Autodesk Inventor part; units mm, degrees
(part 2 of 2)
sketch "Sketch12" plane through (0, 0, 2.55) normal (0, 0, 1) x (1, 0, 0)
  line L0 (1.7095, -0.3755) -> (1.8711, -0.3755)
  line L1 (1.7095, -0.8624) -> (1.7095, -0.3755)
  line L2 (1.7111, -0.0516) -> (1.7111, -0.2119)
  line L3 (1.5448, -0.0527) -> (1.7096, -0.0527)
  line L4 (1.5467, -0.0514) -> (1.5467, -0.2124)
  line L5 (1.5462, -0.2119) -> (1.5462, -0.3755)
  line L6 (1.3838, -0.0514) -> (1.5467, -0.0514)
  line L7 (1.3838, -0.2124) -> (1.3838, -0.0514)
  line L8 (0.8919, -0.3755) -> (0.8919, -0.2124)
  line L9 (1.221, -0.0527) -> (1.0581, -0.0527)
  line L10 (1.056, -0.3755) -> (0.8919, -0.3755)
  line L11 (1.056, -0.2124) -> (1.056, -0.3755)
  line L12 (0.8919, -0.2124) -> (1.056, -0.2124)
  line L13 (1.8711, -0.3755) -> (1.8711, -0.0516)
  line L14 (1.8711, -0.5378) -> (1.8711, -0.3755)
  line L15 (2.0309, -0.5378) -> (1.8711, -0.5378)
  line L16 (1.8711, -0.3755) -> (2.1907, -0.3755)
  line L17 (2.1907, -0.3755) -> (2.1907, -0.5378)
  line L18 (2.1907, -0.3755) -> (2.1907, -0.0491)
  line L19 (2.1907, -0.0491) -> (2.3485, -0.0491)
  line L20 (2.3485, -0.0491) -> (2.3485, -0.3755)
  line L21 (2.3485, -0.3755) -> (2.1907, -0.3755)
  line L22 (1.5467, -0.2124) -> (1.3838, -0.2124)
  line L23 (1.2209, -0.3755) -> (1.057, -0.3755)
  line L24 (1.2209, -0.5378) -> (1.2209, -0.3755)
  line L25 (1.057, -0.7023) -> (0.8965, -0.7023)
  line L26 (1.057, -0.3755) -> (1.057, -0.7023)
  line L27 (1.384, -0.3755) -> (1.384, -0.5378)
  line L28 (1.5462, -0.3755) -> (1.384, -0.3755)
  line L29 (1.7111, -0.2119) -> (1.5462, -0.2119)
  line L30 (1.384, -0.5378) -> (1.2209, -0.5378)
  line L31 (0.8965, -0.7023) -> (0.8965, -1.024)
  line L32 (1.384, -0.7023) -> (1.384, -0.5378)
  line L33 (1.384, -0.5378) -> (1.5462, -0.5378)
  line L34 (1.0586, -1.024) -> (1.0586, -0.8624)
  line L35 (1.5462, -0.5378) -> (1.5462, -0.7023)
  line L36 (1.5462, -0.7023) -> (1.384, -0.7023)
  line L37 (1.0586, -0.8624) -> (1.7095, -0.8624)
  line L38 (0.4096, -0.2124) -> (0.5728, -0.2124)
  line L39 (0.5728, -0.2124) -> (0.5728, -0.3755)
  line L40 (0.5728, -0.0514) -> (0.7344, -0.0514)
  line L41 (0.4096, -0.3755) -> (0.4096, -0.2124)
  line L42 (0.5728, -0.3755) -> (0.4096, -0.3755)
  line L43 (0.4096, -1.0246) -> (0.4096, -0.8624)
  line L44 (0.4096, -0.8624) -> (0.5728, -0.8624)
  line L45 (0.5728, -0.8624) -> (0.5728, -0.7031)
  line L46 (0.5728, -0.7031) -> (0.8961, -0.7031)
  line L47 (0.8961, -0.7031) -> (0.8961, -0.5378)
  line L48 (0.8961, -0.5378) -> (0.4096, -0.5378)
  line L49 (2.1907, -0.5378) -> (2.3485, -0.5378)
  line L50 (2.0309, -0.7023) -> (2.0309, -0.5378)
  line L51 (2.1907, -0.7023) -> (2.0309, -0.7023)
  line L52 (2.3485, -0.5378) -> (2.3485, -1.0249)
  line L53 (2.1907, -1.0249) -> (2.1907, -0.7023)
  line L54 (2.3485, -1.0249) -> (2.1907, -1.0249)
  line L55 (2.0328, -0.8624) -> (2.0328, -1.024)
  line L56 (2.1907, -1.024) -> (2.0328, -1.024)
  line L57 (0.8919, -1.6707) -> (1.056, -1.6707)
  line L58 (1.2181, -1.6707) -> (1.2181, -1.5065)
  line L59 (1.3818, -1.6707) -> (1.2181, -1.6707)
  line L60 (1.2181, -1.5065) -> (1.3818, -1.5065)
  line L61 (1.3818, -1.5065) -> (1.3818, -1.6707)
  line L62 (0.8961, -1.1813) -> (1.2209, -1.1813)
  line L63 (0.8965, -1.024) -> (1.0586, -1.024)
  line L64 (1.2209, -1.1813) -> (1.2209, -1.024)
  line L65 (1.2209, -1.024) -> (1.5448, -1.024)
  line L66 (1.5448, -1.024) -> (1.5448, -1.1813)
  line L67 (1.7075, -1.5065) -> (1.7075, -1.6707)
  line L68 (1.5448, -1.1813) -> (1.7095, -1.1813)
  line L69 (1.7075, -1.6707) -> (1.8711, -1.6707)
  line L70 (1.8711, -1.6707) -> (1.8711, -1.5065)
  line L71 (1.8711, -1.5065) -> (1.7075, -1.5065)
  line L72 (0.8961, -1.3385) -> (1.8711, -1.3385)
  line L73 (1.8711, -1.5065) -> (2.0329, -1.5065)
  line L74 (2.1907, -1.5065) -> (2.0329, -1.5065)
  line L75 (2.3485, -1.6707) -> (2.3485, -1.345)
  line L76 (2.3485, -1.345) -> (2.1907, -1.345)
  line L77 (2.1907, -1.345) -> (2.1907, -1.5065)
  line L78 (1.8711, -1.3385) -> (1.8711, -1.5065)
  line L79 (2.0329, -1.5065) -> (2.0329, -1.3385)
  line L80 (2.0329, -1.3385) -> (1.8711, -1.3385)
  line L81 (1.8711, -1.1813) -> (1.8711, -1.3385)
  line L82 (1.8711, -1.1813) -> (2.1907, -1.1813)
  line L83 (1.7095, -1.1813) -> (1.7095, -0.8624)
  line L84 (1.7095, -0.8624) -> (2.0328, -0.8624)
  line L85 (2.1907, -1.024) -> (2.1907, -1.1813)
  line L86 (0.7344, -1.8284) -> (0.7344, -1.994)
  line L87 (0.7344, -1.994) -> (0.5728, -1.994)
  line L88 (0.5728, -1.8284) -> (0.7344, -1.8284)
  line L89 (0.5728, -1.8284) -> (0.5728, -1.6643)
  line L90 (0.2544, -2.154) -> (0.4096, -2.154)
  line L91 (1.056, -2.1533) -> (0.8919, -2.1533)
  line L92 (0.4096, -2.154) -> (0.4096, -1.8284)
  line L93 (0.5728, -1.994) -> (0.5728, -1.8284)
  line L94 (0.8919, -2.1533) -> (0.8919, -1.6707)
  line L95 (1.056, -1.6707) -> (1.056, -2.1533)
  line L96 (0.4096, -1.8284) -> (0.5728, -1.8284)
  line L97 (1.5448, -2.642) -> (1.5448, -2.1533)
  line L98 (2.0329, -1.5065) -> (2.0329, -1.6707)
  line L99 (1.5448, -2.1533) -> (2.035, -2.1533)
  line L100 (1.3838, -2.8055) -> (1.3838, -1.9925)
  line L101 (1.3838, -1.9925) -> (2.1893, -1.9925)
  line L102 (2.0329, -1.6707) -> (2.3485, -1.6707)
  line L103 (2.035, -2.1533) -> (2.035, -2.642)
  line L104 (2.035, -2.642) -> (1.5448, -2.642)
  line L105 (1.2202, -1.8269) -> (2.3506, -1.8269)
  line L106 (2.1893, -1.9925) -> (2.1893, -2.8055)
  line L107 (2.1893, -2.8055) -> (1.3838, -2.8055)
  line L108 (2.3506, -1.8269) -> (2.3506, -2.9562)
  line L109 (2.3506, -2.9562) -> (1.2202, -2.9562)
  line L110 (1.2202, -2.9562) -> (1.2202, -1.8269)
  line L111 (0.4102, -2.3154) -> (0.5779, -2.3154)
  line L112 (0.7355, -2.3134) -> (1.0581, -2.3134)
  line L113 (1.0581, -2.4698) -> (0.8968, -2.4698)
  line L114 (1.0581, -2.3134) -> (1.0581, -2.4698)
  line L115 (0.5779, -2.4774) -> (0.4102, -2.4774)
  line L116 (0.5779, -2.3154) -> (0.5779, -2.4774)
  line L117 (0.8968, -2.4698) -> (0.8968, -2.6397)
  line L118 (0.8968, -2.6397) -> (0.7355, -2.6397)
  line L119 (0.7355, -2.6397) -> (0.7355, -2.3134)
  line L120 (0.4102, -2.4774) -> (0.4102, -2.3154)
  line L121 (0.4102, -2.6397) -> (0.7355, -2.6397)
  line L122 (0.4102, -2.8009) -> (0.4102, -2.6397)
  line L123 (0.5728, -2.8009) -> (0.4102, -2.8009)
  line L124 (0.7355, -2.9621) -> (0.7355, -2.6397)
  line L125 (0.7355, -2.9621) -> (0.5728, -2.9621)
  line L126 (0.4102, -2.8009) -> (0.255, -2.8009)
  line L127 (0.4102, -2.8009) -> (0.4102, -2.9622)
  line L128 (0.4102, -2.9622) -> (0.0925, -2.9622)
  line L129 (0.5728, -2.9621) -> (0.5728, -2.8009)
  line L130 (0.5728, -1.5065) -> (0.4096, -1.5065)
  line L131 (0.7355, -1.0246) -> (0.4096, -1.0246)
  line L132 (0.4096, -1.1892) -> (0.5728, -1.1892)
  line L133 (0.7355, -1.3385) -> (0.7355, -1.0246)
  line L134 (0.8961, -1.3385) -> (0.8961, -1.1813)
  line L135 (0.8961, -1.3385) -> (0.7355, -1.3385)
  line L136 (0.4096, -1.5065) -> (0.4096, -1.1892)
  line L137 (0.5728, -1.1892) -> (0.5728, -1.5065)
  line L138 (0.7355, -1.5014) -> (0.8961, -1.5014)
  line L139 (0.5728, -1.6643) -> (0.7355, -1.6643)
  line L140 (0.7355, -1.6643) -> (0.7355, -1.5014)
  line L141 (0.8961, -1.5014) -> (0.8961, -1.3385)
  line L142 (-0.0746, -0.8624) -> (-0.2282, -0.8624)
  line L143 (-0.2342, -0.7031) -> (-0.0746, -0.7031)
  line L144 (-0.0746, -0.7031) -> (-0.0746, -0.5378)
  line L145 (-0.2342, -0.5378) -> (-0.2342, -0.7031)
  line L146 (-0.0746, -0.5378) -> (-0.2342, -0.5378)
  line L147 (-0.0746, -0.3755) -> (-0.0746, -0.5378)
  line L148 (-0.5577, -0.7031) -> (-0.3973, -0.7031)
  line L149 (-0.3973, -0.3755) -> (-0.3973, -0.5378)
  line L150 (-0.5577, -0.5378) -> (-0.5577, -0.7031)
  line L151 (-0.3973, -0.5378) -> (-0.5577, -0.5378)
  line L152 (-0.0746, -0.7031) -> (-0.0746, -0.8624)
  line L153 (-0.2282, 0.2745) -> (-0.2282, -0.0491)
  line L154 (-0.2282, -0.0491) -> (-0.0746, -0.0491)
  line L155 (-0.0746, -0.0491) -> (-0.0746, -0.2124)
  line L156 (-0.0746, -0.2124) -> (-0.2282, -0.2124)
  line L157 (-0.2282, -0.2124) -> (-0.2282, -0.0491)
  line L158 (-0.2282, -0.0491) -> (-0.3967, -0.0491)
  line L159 (-0.0746, -0.3755) -> (-0.2357, -0.3755)
  line L160 (-0.5566, 0.1109) -> (-0.3967, 0.1109)
  line L161 (-0.2357, -0.3755) -> (-0.2357, -0.2124)
  line L162 (-0.5566, 0.1109) -> (-0.5566, -0.0491)
  line L163 (-0.2357, -0.2124) -> (-0.5577, -0.2124)
  line L164 (-0.3973, -0.3755) -> (-0.5577, -0.3755)
  line L165 (-0.3967, -0.0491) -> (-0.3967, 0.1109)
  line L166 (0.2535, -1.6707) -> (0.0919, -1.6707)
  line L167 (0.0919, -1.8284) -> (0.2544, -1.8284)
  line L168 (0.2535, -1.5065) -> (0.2535, -1.6707)
  line L169 (0.0919, -1.5065) -> (0.2535, -1.5065)
  line L170 (0.0919, -1.6707) -> (0.0919, -1.5065)
  line L171 (0.0919, -1.1813) -> (0.2507, -1.1813)
  line L172 (-0.2357, -1.8284) -> (-0.0711, -1.8284)
  line L173 (-0.2357, -1.6643) -> (-0.2357, -1.8284)
  line L174 (-0.3973, -1.8284) -> (-0.2342, -1.8284)
  line L175 (-0.3973, -1.8284) -> (-0.3973, -1.6643)
  line L176 (0.0919, -1.3385) -> (0.0919, -1.5064)
  line L177 (0.0919, -1.5064) -> (-0.2342, -1.5064)
  line L178 (-0.0711, -1.3385) -> (0.0919, -1.3385)
  line L179 (-0.3973, -1.6643) -> (-0.2357, -1.6643)
  line L180 (-0.2342, -1.5064) -> (-0.2342, -1.3385)
  line L181 (-0.0711, -1.1813) -> (-0.0711, -1.3385)
  line L182 (-0.3973, -1.1813) -> (-0.0711, -1.1813)
  line L183 (-0.2342, -1.3385) -> (-0.3973, -1.3385)
  line L184 (-0.3973, -1.3385) -> (-0.3973, -1.5014)
  line L185 (-0.7175, -0.3755) -> (-0.7175, -0.7001)
  line L186 (-0.5577, -0.2124) -> (-0.5577, -0.3755)
  line L187 (-0.8836, -0.7001) -> (-0.8836, -0.5378)
  line L188 (-0.8836, -0.3755) -> (-0.7175, -0.3755)
  line L189 (-0.5566, -0.0491) -> (-1.0463, -0.0491)
  line L190 (-0.8836, -0.2124) -> (-0.8836, -0.3755)
  line L191 (-0.8836, -0.5378) -> (-1.0463, -0.5378)
  line L192 (-1.0463, -0.5378) -> (-1.0463, -0.3755)
  line L193 (-1.2063, -0.537) -> (-1.2063, -0.7001)
  line L194 (-1.2063, -0.7001) -> (-1.3676, -0.7001)
  line L195 (-1.3676, -0.537) -> (-1.2063, -0.537)
  line L196 (-1.3676, -0.7001) -> (-1.3676, -0.537)
  line L197 (-1.3676, -0.3755) -> (-1.0463, -0.3755)
  line L198 (-1.3676, -0.3755) -> (-1.3676, -0.2124)
  line L199 (-0.7175, -0.7001) -> (-0.8836, -0.7001)
  line L200 (-0.5566, 0.1109) -> (-0.7175, 0.1109)
  line L201 (-0.5566, 0.2726) -> (-0.5566, 0.1109)
  line L202 (-0.7175, 0.2726) -> (-0.5566, 0.2726)
  line L203 (-0.7175, 0.1109) -> (-0.7175, 0.2726)
  line L204 (-1.0463, -0.0491) -> (-1.0463, -0.2124)
  line L205 (-1.0463, -0.2124) -> (-0.8836, -0.2124)
  line L206 (-1.0463, 0.1109) -> (-0.8836, 0.1109)
  line L207 (-0.8836, 0.1109) -> (-0.8836, 0.4344)
  line L208 (-1.0463, 0.2726) -> (-1.0463, 0.1109)
  line L209 (-1.2069, 0.2726) -> (-1.0463, 0.2726)
  line L210 (-1.2069, 0.1115) -> (-1.2069, 0.2726)
  line L211 (-1.2069, -0.2124) -> (-1.2069, -0.0491)
  line L212 (-1.3676, -0.2124) -> (-1.2069, -0.2124)
  line L213 (-1.3676, -0.0491) -> (-1.3676, 0.1115)
  line L214 (-1.2069, -0.0491) -> (-1.3676, -0.0491)
  line L215 (-1.208, 0.4384) -> (-1.208, 0.2726)
  line L216 (-1.3676, 0.1115) -> (-1.2069, 0.1115)
  line L217 (-1.208, 0.2726) -> (-1.6886, 0.2726)
  line L218 (-1.208, 0.4384) -> (-1.8491, 0.4384)
  line L219 (-1.528, -0.2124) -> (-1.528, -0.0491)
  line L220 (-1.528, -0.0491) -> (-1.6886, -0.0491)
  line L221 (-1.8491, -0.2124) -> (-1.528, -0.2124)
  line L222 (-1.2069, -1.3385) -> (-1.2069, -1.5014)
  line L223 (-1.2069, -1.5014) -> (-1.528, -1.5014)
  line L224 (-1.0463, -1.5014) -> (-1.0463, -1.6643)
  line L225 (-1.528, -1.6643) -> (-1.0463, -1.6643)
  line L226 (-1.528, -1.5014) -> (-1.528, -1.6643)
  line L227 (-1.3682, -1.3385) -> (-1.2069, -1.3385)
  line L228 (-1.0463, -1.3385) -> (-1.0463, -1.1856)
  line L229 (-1.0463, -1.1856) -> (-1.3682, -1.1856)
  line L230 (-1.3682, -1.1856) -> (-1.3682, -1.3385)
  line L231 (-1.528, -1.1856) -> (-1.3682, -1.1856)
  line L232 (-1.3682, -1.1856) -> (-1.3682, -1.024)
  line L233 (-1.3682, -1.024) -> (-1.0463, -1.024)
  line L234 (-1.6826, -0.8624) -> (-1.6826, -1.3385)
  line L235 (-1.528, -0.8624) -> (-1.528, -1.1856)
  line L236 (-1.0463, -0.8624) -> (-1.528, -0.8624)
  line L237 (-1.0463, -1.024) -> (-1.0463, -0.8624)
  line L238 (-0.3973, -0.7031) -> (-0.3973, -1.1813)
  line L239 (-0.7181, -0.8624) -> (-0.8825, -0.8624)
  line L240 (-0.8825, -0.8624) -> (-0.8825, -1.024)
  line L241 (-0.8825, -1.024) -> (-1.0463, -1.024)
  line L242 (-1.0463, -1.1856) -> (-0.7181, -1.1856)
  line L243 (-0.7181, -1.1856) -> (-0.7181, -0.8624)
  line L244 (-1.0463, -1.024) -> (-1.0463, -1.1856)
  line L245 (-2.1731, -0.0514) -> (-2.3367, -0.0514)
  line L246 (-2.3367, -0.0514) -> (-2.3367, 0.1105)
  line L247 (-2.3367, 0.1105) -> (-2.1731, 0.1105)
  line L248 (-2.0121, -0.0491) -> (-1.8491, -0.0491)
  line L249 (-2.1731, 0.1105) -> (-2.1731, -0.0514)
  line L250 (-2.0121, 0.1109) -> (-2.0121, -0.0491)
  line L251 (-1.6886, -0.0491) -> (-1.6886, 0.2726)
  line L252 (-2.0121, 0.2745) -> (-2.174, 0.2745)
  line L253 (-2.174, 0.2745) -> (-2.174, 0.4344)
  line L254 (-2.174, 0.4344) -> (-2.0121, 0.4344)
  line L255 (-2.0121, 0.4344) -> (-2.0121, 0.2745)
  line L256 (-1.8491, 0.4384) -> (-1.8491, 0.1109)
  line L257 (-1.8491, 0.1109) -> (-2.0121, 0.1109)
  line L258 (0.4096, 0.1105) -> (0.4096, 0.2745)
  line L259 (-0.0705, 0.4344) -> (-0.0705, 0.2745)
  line L260 (-0.0705, 0.2745) -> (-0.2282, 0.2745)
  line L261 (-0.0705, 0.4344) -> (0.2555, 0.4344)
  line L262 (0.2555, 0.2745) -> (0.2555, 0.4344)
  line L263 (0.4096, 0.2745) -> (0.2555, 0.2745)
  line L264 (0.4096, 0.4344) -> (0.4096, 0.2745)
  line L265 (-1.8491, -0.0491) -> (-1.8491, -0.2124)
  line L266 (-2.1731, -0.2124) -> (-2.0121, -0.2124)
  line L267 (-2.0121, -0.2124) -> (-2.0121, -0.3755)
  line L268 (-2.1731, -0.3755) -> (-2.1731, -0.2124)
  line L269 (-2.0121, -0.3755) -> (-2.1731, -0.3755)
  line L270 (-2.0099, -0.5378) -> (-2.0099, -0.3755)
  line L271 (-2.0099, -0.3755) -> (-1.6886, -0.3755)
  line L272 (-1.6886, -0.3755) -> (-1.6886, -0.5378)
  line L273 (-2.3339, -0.7001) -> (-2.3339, -0.5378)
  line L274 (-2.0069, -0.7001) -> (-2.3339, -0.7001)
  line L275 (-1.6886, -0.5378) -> (-1.8481, -0.5378)
  line L276 (-2.1731, -0.8624) -> (-2.0069, -0.8624)
  line L277 (-2.0069, -0.8624) -> (-2.0069, -0.7001)
  line L278 (-1.8481, -0.5378) -> (-1.8481, -0.8624)
  line L279 (-1.8481, -0.8624) -> (-1.6826, -0.8624)
  line L280 (-2.1731, -1.1856) -> (-2.1731, -0.8624)
  line L281 (-2.3339, -0.5378) -> (-2.0099, -0.5378)
  line L282 (-0.0746, -0.5378) -> (0.0919, -0.5378)
  line L283 (0.0919, -0.3755) -> (0.0919, -0.5378)
  line L284 (0.4096, -0.5378) -> (0.4096, -0.3755)
  line L285 (0.4096, -0.3755) -> (0.0919, -0.3755)
  line L286 (0.0919, -0.7031) -> (-0.0746, -0.7031)
  line L287 (0.0919, -0.7031) -> (0.0919, -0.8624)
  line L288 (-0.2282, -0.8624) -> (-0.2282, -1.0246)
  line L289 (-0.2282, -1.0246) -> (0.0919, -1.0246)
  line L290 (0.2507, -0.8624) -> (0.0919, -0.8624)
  line L291 (0.0919, -1.0246) -> (0.0919, -1.1813)
  line L292 (0.2507, -1.1813) -> (0.2507, -0.8624)
  line L293 (-1.8457, -1.3385) -> (-1.8457, -1.1856)
  line L294 (-1.6826, -1.3385) -> (-1.8457, -1.3385)
  line L295 (-1.6886, -1.5065) -> (-1.6886, -1.6707)
  line L296 (-2.0121, -1.5065) -> (-1.6886, -1.5065)
  line L297 (-1.6886, -1.6707) -> (-2.0121, -1.6707)
  line L298 (-1.8457, -1.1856) -> (-2.0121, -1.1856)
  line L299 (-2.0121, -1.6707) -> (-2.0121, -1.5065)
  line L300 (-2.0121, -1.1856) -> (-2.0121, -1.3385)
  line L301 (-2.0121, -1.3385) -> (-2.1731, -1.3385)
  line L302 (-2.1731, -1.3385) -> (-2.1731, -1.6643)
  line L303 (-2.3367, -1.1856) -> (-2.1731, -1.1856)
  line L304 (-2.3367, -1.6643) -> (-2.3367, -1.1856)
  line L305 (-2.1731, -1.6643) -> (-2.3367, -1.6643)
  line L306 (-0.7181, -1.3385) -> (-0.7181, -1.1856)
  line L307 (-0.7181, -1.1856) -> (-0.3973, -1.1856)
  line L308 (-0.3973, -1.1856) -> (-0.3973, -1.3385)
  line L309 (-0.7181, -1.5014) -> (-0.7181, -1.3385)
  line L310 (-0.3973, -1.3385) -> (-0.7181, -1.3385)
  line L311 (-0.7175, -1.8284) -> (-0.7175, -1.9925)
  line L312 (-0.7175, -1.9925) -> (-0.5577, -1.9925)
  line L313 (-0.5577, -1.9925) -> (-0.5577, -1.8284)
  line L314 (-0.5577, -1.8284) -> (-0.7175, -1.8284)
  line L315 (-0.3973, -1.9925) -> (-0.3973, -1.8284)
  line L316 (-0.5577, -1.6643) -> (-0.7181, -1.6643)
  line L317 (-0.5577, -1.6643) -> (-0.5577, -1.8284)
  line L318 (-0.5577, -1.8284) -> (-0.3973, -1.8284)
  line L319 (-0.7181, -1.5014) -> (-0.7181, -1.6643)
  line L320 (-0.3973, -1.5014) -> (-0.7181, -1.5014)
  line L321 (-0.7181, -1.8284) -> (-0.7181, -1.6643)
  line L322 (-1.0463, -1.3385) -> (-0.7181, -1.3385)
  line L323 (-1.0463, -1.5014) -> (-0.7181, -1.5014)
  line L324 (-0.7181, -1.6643) -> (-1.0463, -1.6643)
  line L325 (-0.8827, -1.9925) -> (-0.8827, -1.8284)
  line L326 (-0.8827, -1.8284) -> (-0.7181, -1.8284)
  line L327 (-1.0463, -1.6643) -> (-1.0463, -1.9925)
  line L328 (-0.8827, -1.9925) -> (-0.7175, -1.9925)
  line L329 (-0.7175, -1.9925) -> (-0.7175, -2.1533)
  line L330 (-0.7175, -2.1533) -> (-0.8827, -2.1533)
  line L331 (-0.8827, -2.1533) -> (-0.8827, -1.9925)
  line L332 (-1.0463, -1.9925) -> (-0.8827, -1.9925)
  line L333 (-0.3967, -2.1533) -> (-0.3967, -2.3123)
  line L334 (-0.7175, -2.1533) -> (-0.3967, -2.1533)
  line L335 (-0.7175, -2.1533) -> (-0.7175, -2.4774)
  line L336 (-1.0463, -2.3154) -> (-0.8827, -2.3154)
  line L337 (-0.7175, -2.4774) -> (-0.8827, -2.4774)
  line L338 (-0.8827, -2.3154) -> (-0.8827, -2.4774)
  line L339 (-1.0463, -2.4774) -> (-1.0463, -2.3154)
  line L340 (-0.8827, -2.4774) -> (-1.0463, -2.4774)
  line L341 (-0.8827, -2.4774) -> (-0.8827, -2.642)
  line L342 (-2.174, -1.9925) -> (-1.3685, -1.9925)
  line L343 (-2.3376, -1.8269) -> (-1.2073, -1.8269)
  line L344 (-2.013, -2.642) -> (-2.013, -2.1533)
  line L345 (-2.174, -2.8055) -> (-2.174, -1.9925)
  line L346 (-1.5228, -2.1533) -> (-1.5228, -2.642)
  line L347 (-1.5228, -2.642) -> (-2.013, -2.642)
  line L348 (-2.3376, -2.9562) -> (-2.3376, -1.8269)
  line L349 (-1.3685, -1.9925) -> (-1.3685, -2.8055)
  line L350 (-1.3685, -2.8055) -> (-2.174, -2.8055)
  line L351 (-1.2073, -1.8269) -> (-1.2073, -2.9562)
  line L352 (-1.2073, -2.9562) -> (-2.3376, -2.9562)
  line L353 (-2.013, -2.1533) -> (-1.5228, -2.1533)
  line L354 (-1.0463, -2.642) -> (-0.8827, -2.642)
  line L355 (-0.3967, -2.642) -> (-0.3967, -2.8009)
  line L356 (-0.3967, -2.8009) -> (-0.5571, -2.8009)
  line L357 (-0.5571, -2.642) -> (-0.3967, -2.642)
  line L358 (-0.5571, -2.8009) -> (-0.5571, -2.642)
  line L359 (-0.3967, -2.8009) -> (-0.3967, -2.9644)
  line L360 (-0.7175, -2.642) -> (-0.7175, -2.8009)
  line L361 (-0.7175, -2.8009) -> (-0.8827, -2.8009)
  line L362 (-0.8827, -2.642) -> (-0.7175, -2.642)
  line L363 (-0.8827, -2.8009) -> (-0.8827, -2.642)
  line L364 (-0.3967, -2.9644) -> (-1.0463, -2.9644)
  line L365 (-1.0463, -2.9644) -> (-1.0463, -2.642)
  line L366 (-0.0682, -2.3123) -> (-0.0682, -2.154)
  line L367 (-0.0711, -2.154) -> (0.0919, -2.154)
  line L368 (0.255, -2.8009) -> (0.255, -2.4774)
  line L369 (0.0925, -2.9622) -> (0.0925, -2.8009)
  line L370 (-0.3967, -2.3123) -> (-0.2351, -2.3123)
  line L371 (-0.2351, -2.154) -> (-0.2351, -2.3123)
  line L372 (-0.2351, -2.8009) -> (-0.3967, -2.8009)
  line L373 (-0.2351, -2.642) -> (-0.2351, -2.8009)
  line L374 (-0.0705, -2.642) -> (-0.2351, -2.642)
  line L375 (-0.2351, -2.3123) -> (-0.2351, -2.4774)
  line L376 (-0.2351, -2.3123) -> (-0.0682, -2.3123)
  line L377 (-0.0682, -2.154) -> (-0.2351, -2.154)
  line L378 (0.0925, -2.8009) -> (-0.0705, -2.8009)
  line L379 (-0.2351, -2.4774) -> (0.255, -2.4774)
  line L380 (-0.0705, -2.8009) -> (-0.0705, -2.642)
  line L381 (0.2544, -1.8284) -> (0.2544, -2.154)
  line L382 (0.0919, -2.154) -> (0.0919, -1.8284)
  line L383 (-0.0711, -1.8284) -> (-0.0711, -2.154)
  line L384 (-0.2342, -1.8284) -> (-0.2342, -1.9925)
  line L385 (-0.2342, -1.9925) -> (-0.3973, -1.9925)
  line L386 (0.5728, 0.1105) -> (0.4096, 0.1105)
  line L387 (0.4096, 0.2745) -> (0.5728, 0.2745)
  line L388 (0.894, 0.4344) -> (0.5779, 0.4344)
  line L389 (0.735, 0.6007) -> (0.4102, 0.6007)
  line L390 (0.735, 0.6007) -> (0.735, 0.7514)
  line L391 (0.735, 0.7514) -> (0.894, 0.7514)
  line L392 (0.4102, 0.9146) -> (0.894, 0.9146)
  line L393 (0.894, 0.7514) -> (0.894, 0.4344)
  line L394 (1.0581, 0.4344) -> (1.0581, 0.9141)
  line L395 (1.0581, 0.4344) -> (1.5448, 0.4344)
  line L396 (1.2202, 0.6007) -> (1.2202, 0.7514)
  line L397 (1.3818, 0.6007) -> (1.2202, 0.6007)
  line L398 (1.2202, 0.7514) -> (1.3818, 0.7514)
  line L399 (1.3818, 0.7514) -> (1.3818, 0.6007)
  line L400 (0.5728, 1.239) -> (0.5728, 1.0768)
  line L401 (0.894, 1.0768) -> (1.3838, 1.0768)
  line L402 (0.894, 0.9146) -> (0.894, 1.0768)
  line L403 (0.7345, 1.0768) -> (0.7345, 1.239)
  line L404 (0.7345, 1.239) -> (1.2209, 1.239)
  line L405 (0.7345, 1.4023) -> (0.7345, 1.239)
  line L406 (0.5728, 1.0768) -> (0.7345, 1.0768)
  line L407 (0.7345, 1.239) -> (0.5728, 1.239)
  line L408 (0.5728, 1.4023) -> (0.7345, 1.4023)
  line L409 (0.5728, 1.5644) -> (0.5728, 1.4023)
  line L410 (1.2209, 1.5644) -> (0.5728, 1.5644)
  line L411 (1.2209, 1.239) -> (1.2209, 1.5644)
  line L412 (0.0919, 1.5644) -> (0.2507, 1.5644)
  line L413 (0.0919, 1.4017) -> (0.0919, 1.5644)
  line L414 (0.2507, 1.239) -> (0.2507, 1.5644)
  line L415 (-0.0733, 1.5644) -> (-0.0733, 1.4017)
  line L416 (0.2507, 1.0768) -> (0.2507, 1.239)
  line L417 (-0.2353, 1.5644) -> (-0.0733, 1.5644)
  line L418 (0.2507, 1.239) -> (-0.2353, 1.239)
  line L419 (-0.2353, 1.239) -> (-0.2353, 1.5644)
  line L420 (0.2507, 1.73) -> (-0.3973, 1.73)
  line L421 (-0.3973, 1.73) -> (-0.3973, 1.0768)
  line L422 (-0.0733, 1.4017) -> (0.0919, 1.4017)
  line L423 (0.7344, 0.1105) -> (0.5728, 0.1105)
  line L424 (0.5728, 0.2745) -> (0.5728, 0.1105)
  line L425 (0.894, 0.2745) -> (0.894, 0.1115)
  line L426 (0.5779, 0.2745) -> (0.894, 0.2745)
  line L427 (0.5779, 0.4344) -> (0.5779, 0.2745)
  line L428 (1.0581, 0.2745) -> (1.3838, 0.2745)
  line L429 (1.3838, 0.2745) -> (1.3838, 0.1115)
  line L430 (1.3838, 0.1115) -> (1.5448, 0.1115)
  line L431 (1.5448, 0.1115) -> (1.5448, -0.0527)
  line L432 (1.0581, 0.1115) -> (1.0581, 0.2745)
  line L433 (1.0581, 0.1115) -> (1.221, 0.1115)
  line L434 (1.221, 0.1115) -> (1.221, -0.0527)
  line L435 (1.0581, -0.0527) -> (1.0581, 0.1115)
  line L436 (0.7344, -0.0514) -> (0.7344, 0.1105)
  line L437 (0.5728, 0.1105) -> (0.5728, -0.0514)
  line L438 (0.894, 0.1115) -> (1.0581, 0.1115)
  line L439 (1.3838, 1.0768) -> (1.3838, 1.2402)
  line L440 (1.5462, 1.4023) -> (1.5462, 1.5644)
  line L441 (1.5448, 0.9141) -> (1.0581, 0.9141)
  line L442 (1.5467, 1.2402) -> (1.5467, 1.0768)
  line L443 (1.5462, 1.4023) -> (1.7111, 1.4023)
  line L444 (1.7096, 1.0768) -> (1.7096, 0.9141)
  line L445 (1.3838, 1.2402) -> (1.5467, 1.2402)
  line L446 (1.7096, 0.2745) -> (1.7096, -0.0527)
  line L447 (1.8711, -0.0516) -> (1.7111, -0.0516)
  line L448 (1.8711, 0.2745) -> (1.8711, 0.1117)
  line L449 (2.0328, 0.1117) -> (2.0328, -0.0491)
  line L450 (2.0328, -0.0491) -> (2.1907, -0.0491)
  line L451 (2.1907, -0.0491) -> (2.1907, 0.2745)
  line L452 (2.1907, 0.2745) -> (1.8711, 0.2745)
  line L453 (1.8711, 0.1117) -> (2.0328, 0.1117)
  line L454 (1.5467, 1.0768) -> (1.7096, 1.0768)
  line L455 (2.0302, 0.4343) -> (2.1838, 0.4343)
  line L456 (1.8711, 0.2745) -> (1.7096, 0.2745)
  line L457 (1.8711, 0.6015) -> (1.8711, 0.2745)
  line L458 (2.1838, 0.4343) -> (2.1838, 0.5928)
  line L459 (2.0302, 0.6015) -> (2.0302, 0.4343)
  line L460 (2.0302, 0.6015) -> (1.8711, 0.6015)
  line L461 (2.1838, 0.7546) -> (2.1838, 0.5928)
  line L462 (1.7096, 0.7514) -> (1.8711, 0.7514)
  line L463 (1.5448, 0.9141) -> (1.5448, 0.4344)
  line L464 (1.8711, 0.9141) -> (2.0302, 0.9141)
  line L465 (1.8711, 0.7514) -> (1.8711, 0.9141)
  line L466 (1.7096, 0.7514) -> (1.7096, 0.9141)
  line L467 (2.0302, 0.9141) -> (2.0302, 0.7546)
  line L468 (2.0302, 0.7546) -> (2.1838, 0.7546)
  line L469 (0.4102, 0.9141) -> (0.4102, 1.0768)
  line L470 (0.4102, 1.0768) -> (0.2507, 1.0768)
  line L471 (0.2555, 0.4344) -> (0.4096, 0.4344)
  line L472 (0.2555, 0.4344) -> (0.2555, 0.6023)
  line L473 (0.4102, 0.6007) -> (0.4102, 0.9146)
  line L474 (-0.0702, 0.6023) -> (0.2555, 0.6023)
  line L475 (-0.0702, 0.7535) -> (-0.0702, 0.6023)
  line L476 (-0.0733, 0.9141) -> (0.4102, 0.9141)
  line L477 (-0.2351, 0.7535) -> (-0.0702, 0.7535)
  line L478 (-0.2351, 0.6023) -> (-0.2351, 0.7535)
  line L479 (-0.3946, 0.6023) -> (-0.2351, 0.6023)
  line L480 (-0.0733, 1.0768) -> (-0.0733, 0.9141)
  line L481 (-0.3973, 1.0768) -> (-0.0733, 1.0768)
  line L482 (1.7111, 1.0832) -> (1.7111, 1.4023)
  line L483 (2.0309, 1.2402) -> (2.0309, 1.0832)
  line L484 (2.0309, 1.0832) -> (1.7111, 1.0832)
  line L485 (1.8711, 1.4023) -> (1.8711, 1.2402)
  line L486 (1.7111, 1.73) -> (1.7111, 1.5644)
  line L487 (1.8711, 1.2402) -> (2.0309, 1.2402)
  line L488 (2.1907, 1.4023) -> (1.8711, 1.4023)
  line L489 (1.7111, 1.5644) -> (2.3485, 1.5644)
  line L490 (2.3485, 1.2402) -> (2.1907, 1.2402)
  line L491 (2.3485, 1.5644) -> (2.3485, 1.2402)
  line L492 (2.1907, 1.2402) -> (2.1907, 1.4023)
  line L493 (0.2507, 1.5644) -> (0.2507, 1.73)
  line L494 (0.4102, 1.239) -> (0.2507, 1.239)
  line L495 (0.4102, 1.5644) -> (0.4102, 1.239)
  line L496 (0.2507, 1.5644) -> (0.4102, 1.5644)
  line L497 (0.4102, 1.73) -> (0.4102, 1.5644)
  line L498 (0.5728, 1.5644) -> (0.5728, 1.73)
  line L499 (0.5728, 1.73) -> (0.4102, 1.73)
  line L500 (0.4102, 1.5644) -> (0.5728, 1.5644)
  line L501 (-0.8836, 0.4344) -> (-1.0463, 0.4344)
  line L502 (-1.0463, 0.4344) -> (-1.0463, 0.9141)
  line L503 (-0.8827, 0.6023) -> (-0.7175, 0.6023)
  line L504 (-0.7175, 0.6023) -> (-0.7175, 0.7514)
  line L505 (-0.7175, 0.7514) -> (-0.8827, 0.7514)
  line L506 (-0.5544, 0.7514) -> (-0.7175, 0.7514)
  line L507 (-0.5544, 0.7514) -> (-0.5544, 0.9141)
  line L508 (-0.7175, 0.7514) -> (-0.7175, 1.0768)
  line L509 (-0.3946, 0.9141) -> (-0.3946, 0.6023)
  line L510 (-0.5544, 0.9141) -> (-0.3946, 0.9141)
  line L511 (-1.0463, 1.0768) -> (-1.0463, 1.2402)
  line L512 (-1.0463, 1.4036) -> (-1.0463, 1.2402)
  line L513 (-0.8827, 0.7514) -> (-0.8827, 0.6023)
  line L514 (-0.7175, 1.0768) -> (-0.5566, 1.0768)
  line L515 (-0.8836, 0.9141) -> (-0.8836, 1.0768)
  line L516 (-1.0463, 0.9141) -> (-0.8836, 0.9141)
  line L517 (-0.5566, 1.0768) -> (-0.5566, 1.4036)
  line L518 (-0.7175, 1.2402) -> (-0.8827, 1.2402)
  line L519 (-0.7175, 1.4036) -> (-0.7175, 1.2402)
  line L520 (-0.8836, 1.0768) -> (-1.0463, 1.0768)
  line L521 (-0.5566, 1.4036) -> (-0.5566, 1.5644)
  line L522 (-0.8827, 1.4036) -> (-0.7175, 1.4036)
  line L523 (-0.8827, 1.5644) -> (-0.5566, 1.5644)
  line L524 (-0.8827, 1.4036) -> (-0.8827, 1.5644)
  line L525 (-1.0463, 1.4036) -> (-0.8827, 1.4036)
  line L526 (-0.8827, 1.2402) -> (-0.8827, 1.4036)
  line L527 (-0.8836, 1.5644) -> (-1.0463, 1.5644)
  line L528 (-0.8836, 1.73) -> (-0.8836, 1.5644)
  line L529 (-1.0463, 1.73) -> (-0.8836, 1.73)
  line L530 (-1.0463, 1.5644) -> (-1.0463, 1.73)
  line L531 (1.2209, 1.5644) -> (1.2209, 1.73)
  line L532 (1.5462, 1.5644) -> (1.2209, 1.5644)
  line L533 (1.2209, 1.73) -> (1.7111, 1.73)
  line L534 (1.2374, 2.5034) -> (1.3667, 2.5034)
  line L535 (1.3667, 2.5034) -> (1.3667, 2.2334)
  line L536 (1.3667, 2.2334) -> (1.2374, 2.2334)
  line L537 (1.2374, 2.6356) -> (1.2374, 2.5034)
  line L538 (0.8281, 2.6356) -> (1.2374, 2.6356)
  line L539 (1.2374, 2.5034) -> (0.8281, 2.5034)
  line L540 (1.2374, 2.2334) -> (1.2374, 2.5034)
  line L541 (1.2374, 2.2334) -> (0.8281, 2.2334)
  line L542 (1.2374, 2.109) -> (1.2374, 2.2334)
  line L543 (0.8281, 2.109) -> (1.2374, 2.109)
  line L544 (0.8281, 2.6356) -> (0.6989, 2.6356)
  line L545 (0.8281, 2.5034) -> (0.8281, 2.6356)
  line L546 (0.8281, 2.2334) -> (0.8281, 2.109)
  line L547 (0.8281, 2.5034) -> (0.8281, 2.2334)
  line L548 (0.6989, 2.2334) -> (0.6989, 2.5034)
  line L549 (0.6989, 2.5034) -> (0.8281, 2.5034)
  line L550 (0.5437, 2.2334) -> (0.5437, 2.109)
  line L551 (0.8281, 2.2334) -> (0.6989, 2.2334)
  line L552 (-1.5219, 1.4036) -> (-1.5219, 0.9149)
  line L553 (-1.3676, 1.5644) -> (-1.3676, 0.7514)
  line L554 (-1.5219, 0.9149) -> (-2.0121, 0.9149)
  line L555 (-2.0121, 1.4036) -> (-1.5219, 1.4036)
  line L556 (-2.0121, 0.9149) -> (-2.0121, 1.4036)
  line L557 (-1.2063, 1.73) -> (-1.2063, 0.6007)
  line L558 (-1.3676, 0.7514) -> (-2.1731, 0.7514)
  line L559 (-2.1731, 1.5644) -> (-1.3676, 1.5644)
  line L560 (-1.2063, 0.6007) -> (-2.3367, 0.6007)
  line L561 (-2.3367, 0.6007) -> (-2.1731, 0.6007)
  line L562 (-2.1731, 0.7514) -> (-2.1731, 1.5644)
  line L563 (-2.3367, 0.6007) -> (-2.3367, 1.73)
  line L564 (-2.3367, 1.73) -> (-1.2063, 1.73)
  line L565 (-1.3676, 2.2334) -> (-1.5014, 2.2334)
  line L566 (-1.5014, 2.2334) -> (-1.5014, 2.109)
  line L567 (-1.0999, 2.2334) -> (-1.2274, 2.2334)
  line L568 (-1.0999, 2.109) -> (-1.0999, 2.2334)
  line L569 (-1.5014, 2.109) -> (-1.0999, 2.109)
  line L570 (-0.1284, 2.7689) -> (-0.1284, 2.9022)
  line L571 (0.0138, 2.7689) -> (-0.1284, 2.7689)
  line L572 (-0.1284, 2.9022) -> (0.0138, 2.9022)
  line L573 (0.0138, 2.9022) -> (0.0138, 2.7689)
  line L574 (0.0138, 3.0367) -> (0.0138, 2.9022)
  line L575 (0.2766, 2.5034) -> (0.143, 2.5034)
  line L576 (0.2766, 2.6356) -> (0.2766, 2.5034)
  line L577 (0.4102, 2.6356) -> (0.4102, 2.9022)
  line L578 (0.4102, 2.6356) -> (0.2766, 2.6356)
  line L579 (0.2766, 2.5034) -> (0.4102, 2.5034)
  line L580 (0.4102, 2.5034) -> (0.4102, 2.6356)
  line L581 (0.0138, 2.9022) -> (0.4102, 2.9022)
  line L582 (0.4102, 2.9022) -> (0.4102, 3.0367)
  line L583 (0.4102, 3.0367) -> (0.0138, 3.0367)
  line L584 (0.8281, 2.9022) -> (0.8281, 2.6356)
  line L585 (0.6989, 2.9022) -> (0.8281, 2.9022)
  line L586 (0.6989, 2.6356) -> (0.6989, 2.9022)
  line L587 (0.5437, 2.9022) -> (0.5437, 2.6356)
  line L588 (0.4102, 2.9022) -> (0.5437, 2.9022)
  line L589 (0.5437, 2.6356) -> (0.4102, 2.6356)
  line L590 (-0.2763, 3.0367) -> (-0.2763, 2.109)
  line L591 (0.2766, 2.3684) -> (0.2766, 2.5034)
  line L592 (0.143, 2.3684) -> (0.2766, 2.3684)
  line L593 (0.5437, 2.109) -> (-0.1284, 2.109)
  line L594 (-0.1284, 2.2334) -> (0.5437, 2.2334)
  line L595 (0.143, 2.2334) -> (0.143, 2.3684)
  line L596 (0.143, 2.5034) -> (0.143, 2.3684)
  line L597 (0.0138, 2.2334) -> (0.143, 2.2334)
  line L598 (0.143, 2.3684) -> (0.0138, 2.3684)
  line L599 (0.0138, 2.3684) -> (0.0138, 2.2334)
  line L600 (-0.1284, 2.109) -> (-0.1284, 2.2334)
  line L601 (-0.4137, 2.109) -> (-0.4137, 2.7689)
  line L602 (-0.2763, 2.109) -> (-0.4137, 2.109)
  line L603 (-0.5459, 2.7689) -> (-0.5459, 2.5034)
  line L604 (-0.5459, 2.5034) -> (-0.6808, 2.5034)
  line L605 (-0.4137, 2.9022) -> (-0.4137, 3.0367)
  line L606 (-0.5459, 2.7689) -> (-0.4137, 2.7689)
  line L607 (-0.5459, 2.9022) -> (-0.5459, 2.7689)
  line L608 (-0.4137, 2.9022) -> (-0.5459, 2.9022)
  line L609 (-0.6808, 2.7689) -> (-0.5459, 2.7689)
  line L610 (-0.4137, 3.0367) -> (-0.2763, 3.0367)
  line L611 (-0.9535, 3.0367) -> (-0.8137, 3.0367)
  line L612 (-0.9535, 2.109) -> (-0.9535, 3.0367)
  line L613 (-0.8137, 3.0367) -> (-0.8137, 2.9022)
  line L614 (-0.6808, 2.9022) -> (-0.6808, 2.7689)
  line L615 (-0.8137, 2.9022) -> (-0.6808, 2.9022)
  line L616 (-0.6808, 2.5034) -> (-0.6808, 2.7689)
  line L617 (-0.8137, 2.109) -> (-0.9535, 2.109)
  line L618 (-0.8137, 2.7689) -> (-0.8137, 2.109)
  line L619 (-0.6808, 2.7689) -> (-0.8137, 2.7689)
  line L620 (-1.6638, 3.0367) -> (-1.6638, 2.9022)
  line L621 (-1.0999, 2.9022) -> (-1.2274, 2.9022)
  line L622 (-1.2274, 2.9022) -> (-1.2274, 2.2334)
  line L623 (-1.0999, 3.0367) -> (-1.0999, 2.9022)
  line L624 (-1.3676, 2.2334) -> (-1.3676, 2.9022)
  line L625 (-1.6638, 2.5034) -> (-1.6638, 2.2334)
  line L626 (-1.6638, 2.2334) -> (-1.7982, 2.2334)
  line L627 (-1.7982, 2.5034) -> (-1.6638, 2.5034)
  line L628 (-1.3676, 2.9022) -> (-1.5014, 2.9022)
  line L629 (-1.5014, 2.9022) -> (-1.5014, 3.0367)
  line L630 (-1.5014, 3.0367) -> (-1.0999, 3.0367)
  line L631 (-2.1927, 2.6356) -> (-2.1927, 2.9022)
  line L632 (-2.1927, 2.9022) -> (-2.1927, 3.0367)
  line L633 (-2.1927, 3.0367) -> (-1.6638, 3.0367)
  line L634 (-1.6638, 2.9022) -> (-2.1927, 2.9022)
  line L635 (-1.7982, 2.2334) -> (-1.7982, 2.5034)
  line L636 (-1.7982, 2.6356) -> (-1.7982, 2.5034)
  line L637 (-1.7982, 2.109) -> (-1.7982, 2.2334)
  line L638 (-2.1927, 2.5034) -> (-2.1927, 2.6356)
  line L639 (-2.1927, 2.6356) -> (-1.7982, 2.6356)
  line L640 (-1.7982, 2.2334) -> (-2.3249, 2.2334)
  line L641 (-2.3249, 2.109) -> (-1.7982, 2.109)
  line L642 (-2.3249, 2.2334) -> (-2.3249, 2.109)
  line L643 (-2.3249, 2.6356) -> (-2.1927, 2.6356)
  line L644 (-2.1927, 2.9022) -> (-2.3249, 2.9022)
  line L645 (-2.3249, 2.9022) -> (-2.3249, 2.6356)
  line L646 (-1.7982, 2.5034) -> (-2.1927, 2.5034)
  line L647 (1.7894, 2.5034) -> (1.7894, 2.7689)
  line L648 (1.9243, 2.5034) -> (1.7894, 2.5034)
  line L649 (1.9243, 2.7689) -> (1.9243, 2.5034)
  line L650 (1.5167, 2.109) -> (1.5167, 3.0367)
  line L651 (2.1939, 3.0367) -> (2.1939, 2.109)
  line L652 (2.0566, 2.109) -> (2.0566, 2.7689)
  line L653 (1.6566, 2.7689) -> (1.6566, 2.109)
  line L654 (1.6566, 2.109) -> (1.5167, 2.109)
  line L655 (2.1939, 2.109) -> (2.0566, 2.109)
  line L656 (1.9243, 2.7689) -> (2.0566, 2.7689)
  line L657 (1.7894, 2.7689) -> (1.9243, 2.7689)
  line L658 (1.9243, 2.9022) -> (1.9243, 2.7689)
  line L659 (2.0566, 2.9022) -> (1.9243, 2.9022)
  line L660 (2.0566, 3.0367) -> (2.1939, 3.0367)
  line L661 (1.7894, 2.7689) -> (1.6566, 2.7689)
  line L662 (1.7894, 2.9022) -> (1.7894, 2.7689)
  line L663 (2.0566, 2.9022) -> (2.0566, 3.0367)
  line L664 (1.6566, 2.9022) -> (1.7894, 2.9022)
  line L665 (1.5167, 3.0367) -> (1.6566, 3.0367)
  line L666 (1.2374, 2.9022) -> (1.3667, 2.9022)
  line L667 (1.2374, 2.6356) -> (1.2374, 2.9022)
  line L668 (1.3667, 2.6356) -> (1.2374, 2.6356)
  line L669 (1.3667, 2.9022) -> (1.3667, 2.6356)
  line L670 (0.8281, 2.9022) -> (1.2374, 2.9022)
  line L671 (0.8281, 3.0367) -> (0.8281, 2.9022)
  line L672 (1.2374, 3.0367) -> (0.8281, 3.0367)
  line L673 (1.2374, 2.9022) -> (1.2374, 3.0367)
  line L674 (1.6566, 3.0367) -> (1.6566, 2.9022)
  point P0 (0, 0)
  constraints: 1350 end point, 299 perpendicular, 194 point on line, 175 parallel, 105 horizontal, 19 vertical
extrude "Extrusion16" add sketch "Sketch12" along normal blind 0.01 contours L1 L37 L34 L63 L31 L25 L26 L23 L24 L30 L27 L28 L5 L29 L2 L447 L13 L0 | L16 L17 L49 L52 L54 L53 L51 L50 L15 L14 | L84 L55 L56 L85 L82 L81 L72 L134 L62 L64 L65 L66 L68 L83 | L74 L77 L76 L75 L102 L98 | L70 L69 L67 L71 | L80 L79 L73 L78 | L88 L86 L87 L93 | L119 L112 L114 L113 L117 L118 | L122 L121 L124 L125 L129 L123 | L340 L339 L336 L338 | L41 L38 L39 L42 | L10 L8 L12 L11 | L433 L434 L9 L435 | L531 L533 L486 L489 L491 L490 L492 L488 L485 L487 L483 L484 L482 L443 L440 L532 | L403 L406 L400 L407 | L410 L411 L404 L405 L408 L409 | L497 L499 L498 L500 | L476 L480 L481 L421 L420 L493 L412 L413 L422 L415 L417 L419 L418 L416 L470 L469 | L18 L19 L20 L21 | L3 L431 L430 L429 L428 L432 L438 L425 L426 L427 L388 L393 L391 L390 L389 L473 L392 L402 L401 L439 L445 L442 L454 L444 L466 L462 L465 L464 L467 L468 L461 L458 L455 L459 L460 L457 L456 L446 | L450 L449 L453 L448 L452 L451 | L4 L22 L7 L6 | L46 L45 L44 L43 L131 L133 L135 L141 L138 L140 L139 L89 L96 L92 L90 L381 L167 L382 L367 L383 L172 L173 L179 L175 L318 L317 L316 L319 L320 L184 L183 L180 L177 L176 L178 L181 L182 L238 L148 L150 L151 L149 L164 L186 L163 L161 L159 L147 L282 L283 L285 L284 L48 L47 | L366 L376 L371 L377 L367 | L414 L496 L495 L494 | L375 L379 L368 L126 L127 L128 L369 L378 L380 L374 L373 L372 L359 L364 L365 L354 L341 L337 L335 L334 L333 L370 | L384 L385 L315 L174 | L330 L331 L328 L329 | L313 L312 L311 L314 | L326 L325 L332 L327 L324 L321 | L323 L224 L225 L226 L223 L222 L227 L230 L229 L228 L322 L309 | L310 L306 L307 L308 | L242 L244 L241 L240 L239 L243 | L231 L235 L236 L237 L233 L232 | L437 L423 L436 L40 | L154 L155 L156 L157 | L217 L251 L220 L219 L221 L265 L248 L250 L257 L256 L218 L215 | L527 L530 L529 L528 | L261 L259 L260 L153 L158 L165 L160 L162 L189 L204 L205 L190 L188 L185 L199 L187 L191 L192 L197 L198 L212 L211 L214 L213 L216 L210 L209 L208 L206 L207 L501 L502 L516 L515 L520 L511 L512 L525 L524 L523 L521 L517 L514 L508 L506 L507 L510 L509 L479 L478 L477 L475 L474 L472 | L263 L262 L471 L264 | L386 L258 L387 L424 | L57 L95 L91 L94 | L58 L60 L61 L59 | L97 L99 L103 L104 | L105 L108 L109 L110 | L111 L116 L115 L120 | L193 L194 L196 L195 | L234 L294 L293 L298 L300 L301 L302 L305 L304 L303 L280 L276 L277 L274 L273 L281 L270 L271 L272 L275 L278 L279 | L245 L246 L247 L249 | L252 L253 L254 L255 | L266 L267 L269 L268 | L295 L297 L299 L296 | L343 L351 L352 L348 | L344 L353 L346 L347 | L396 L398 L399 L397 | L539 L545 L538 L537 | L534 L535 L536 L540 | L667 L666 L669 L668 | L547 L551 L548 L549 | L542 L543 L546 L541 | L544 L586 L585 L584 | L670 L671 L672 L673 | L573 L571 L570 L572 | L581 L574 L583 L582 | L577 L588 L587 L589 | L576 L578 L580 L579 | L596 L575 L591 L592 | L550 L593 L600 L594 | L594 L599 L598 L595 | L552 L554 L556 L555 | L557 L560 L563 L564 | L624 L628 L629 L630 L623 L621 L622 L567 L568 L569 L566 L565 | L619 L618 L617 L612 L611 L613 L615 L614 | L603 L604 L616 L609 | L590 L602 L601 L606 L607 L608 L605 L610 | L637 L641 L642 L640 | L627 L625 L626 L635 | L639 L636 L646 L638 | L631 L643 L645 L644 | L620 L634 L632 L633 | L661 L653 L654 L650 L665 L674 L664 L662 | L658 L659 L663 L660 L651 L655 L652 L656 | L647 L657 L649 L648
